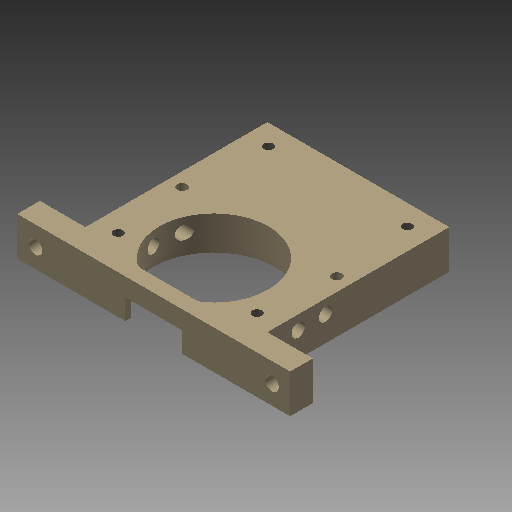
# Autodesk Inventor part: Lichtschranke3
Saved by Autodesk Inventor 2018 (Build 220112000, 112)
## iProperties
Created: 2012-08-13
Part Number: Lichtschranke3
Material: PMMA Plastic
Document SubType Name: Modeling
Designer: Neef
Mass: 81.8294 g
Surface Area: 151.28 cm^2
Volume: 68.88 cm^3
Density: 1.188 g/cm^3
Appearance: Wheat
Author: neef
Autodesk Inventor part; units mm, degrees
ref_plane "YZ Plane" through (0, 0, 0) normal (1, 0, 0) x (0, 1, 0)
ref_plane "XZ Plane" through (0, 0, 0) normal (0, 1, 0) x (-1, 0, 0)
ref_plane "XY Plane" through (0, 0, 0) normal (0, 0, 1) x (1, 0, 0)
sketch "Skizze1" plane through (0, 0, 0) normal (0, 0, 1) x (1, 0, 0)
  line L0 (-40, 45) -> (40, 45)
  line L1 (40, 45) -> (40, -45)
  line L2 (40, -45) -> (-40, -45)
  line L3 (-40, -45) -> (-40, 45)
  line L4 (0, 63) -> (0, -63) projected
  line L5 (-56, 0) -> (56, 0) projected
  point P0 (0, 0)
  point P1 (0, 45)
  point P2 (-40, 0)
  dimension "d0" = 80
  dimension "d1" = 90
  constraints: 8 end point, 2 midpoint, 2 parallel, 2 point on line, 1 horizontal, 1 perpendicular
  measures "d0" distance of L0.start L0.end
  measures "d1" distance of L2.end L0.start
extrude "Extrusion1" add sketch "Skizze1" along normal blind 12
sketch "Skizze2" plane through (0, 0, 0) normal (0, 0, -1) x (-1, 0, 0)
  circle A0 centre (0, -13) radius 5 projected
  circle A1 centre (0, -13) radius 12.5
  point P0 (0, 0)
  dimension "d4" = 25
  constraints: 1 centre point, 1 coincident
  measures "d4" diameter of A1
extrude "Extrusion2" cut sketch "Skizze2" against normal up to surface (12 mm away) contours A0 | A1
sketch "Skizze4" plane through (0, 0, 0) normal (0, 0, -1) x (-1, 0, 0)
  circle A0 centre (30.5, -29.5) radius 2.6 projected
  circle A1 centre (-30.5, -29.5) radius 2.6 projected
  circle A2 centre (30.5, 36.5) radius 2.6 projected
  circle A3 centre (-30.5, 36.5) radius 2.6 projected
  circle A4 centre (-30.5, 36.5) radius 4
  circle A5 centre (30.5, 36.5) radius 4
  circle A6 centre (30.5, -29.5) radius 4
  circle A7 centre (-30.5, -29.5) radius 4
  point P0 (0, 0)
  dimension "d14" = 8
  dimension "d15" = 8
  dimension "d16" = 8
  dimension "d17" = 8
  constraints: 4 centre point, 4 coincident
  measures "d14" diameter of A4
  measures "d15" diameter of A5
  measures "d16" diameter of A6
  measures "d17" diameter of A7
extrude "Extrusion3" cut sketch "Skizze4" against normal blind 4.1
sketch "Skizze6" plane through (0, 0, 0) normal (0, 0, -1) x (-1, 0, 0)
  circle A0 centre (0, -13) radius 12.5 projected
  line L0 (40, 45) -> (40, -45) projected
  arc A1 (0, -29.5) -> (0, 3.5) centre (0, -13) ccw
  arc A2 (19.5, -13) -> (0, 6.5) centre (0, -13) ccw
  line L1 (23.5, -20.5) -> (21, -20.5)
  line L2 (19.5, -13) -> (19.5, -19)
  line L3 (0, 14.2636) -> (0, -32.5)
  line L4 (0, -32.5) -> (20.7123, -32.5)
  line L5 (23.5, -27.0294) -> (23.5, -20.5)
  arc A3 (19.5, -19) -> (21, -20.5) centre (21, -19) ccw
  circle A4 centre (0, -18.5) radius 25 construction
  arc A5 (20.7123, -32.5) -> (23.5, -27.0294) centre (0, -18.5) ccw
  point P0 (0, 0)
  dimension "d22" = 33
  dimension "d23" = 39
  dimension "d24" = 7.5
  dimension "d25" = 19.5
  dimension "d27" = 19.5
  dimension "d28" = 23.5
  dimension "d29" = 1.5
  dimension "d70" = 50
  constraints: 10 end point, 10 point on circle, 5 centre point, 4 point on line, 4 tangent, 3 perpendicular, 2 coincident, 2 parallel, 1 concentric
  measures "d22" diameter of A1
  measures "d23" diameter of A2
  measures "d24" distance from line of A2.centre L1
  measures "d25" distance from line of A0.centre L2
  measures "d27" distance from line of A0.centre L4
  measures "d28" distance from line of A0.centre L5
  measures "d29" radius of A3
  measures "d70" diameter of A4
extrude "Extrusion4" add sketch "Skizze6" along normal blind 5 contours L3 A2 L2 A3 L1 L5 A5 L4 A1
mirror "Spiegeln1" about plane through (0, 3.5, 0) normal (1, 0, 0) of "Extrusion4"
chamfer "Fase1" distance 2 angle 45 1 edges at (0, -29.5, -5)
sketch "Skizze8" plane through (40, -45, 0) normal (1, 0, 0) x (0, 0, -1)
  line L0 (0, 19.5) -> (-12, 19.5) projected
  point P0 (0, 45)
  point P1 (-6, 23.5)
  point P2 (-6, 35.5)
  dimension "d45" = 12
  dimension "d46" = 4
  measures "d45" distance of point (-6, 35.5) point (-6, 23.5)
  measures "d46" distance from line of point (-6, 23.5) L0
hole "Bohrung3" at (40, -21.5, 6) at (40, -9.5, 6) direction (-1, 0, 0) diameter 5.9 end through all
sketch "Skizze11" plane through (0, 0, -5) normal (0, 0, -1) x (-1, 0, 0)
  arc A0 (19.5, -13) -> (-19.5, -13) centre (0, -13) ccw projected
  circle A1 centre (0, -18.5) radius 25
  circle A2 centre (0, -18.5) radius 27
  point P0 (0, 0)
  dimension "d60" = 50
  dimension "d61" = 54
  constraints: 2 centre point, 1 coincident, 1 tangent
  measures "d60" diameter of A1
  measures "d61" diameter of A2
sketch "Skizze12" plane through (0, 0, 0) normal (0, 0, -1) x (-1, 0, 0)
  line L0 (-12.5, -47.3071) -> (12.5, -47.3071)
  line L1 (12.5, -47.3071) -> (12.5, -42)
  line L2 (10.5, -40) -> (-10.5, -40)
  line L3 (-12.5, -42) -> (-12.5, -47.3071)
  line L4 (40, -45) -> (-40, -45) projected
  arc A0 (-10.5, -40) -> (-12.5, -42) centre (-10.5, -42) ccw
  arc A1 (12.5, -42) -> (10.5, -40) centre (10.5, -42) ccw
  point P0 (0, -18.5)
  point P1 (0, 0)
  point P2 (12.5, -40)
  point P3 (-12.5, -40)
  point P4 (5.172, -45)
  dimension "d64" = 25
  dimension "d65" = 12.5
  dimension "d66" = 5
  dimension "d67" = 2
  constraints: 8 end point, 4 point on circle, 4 point on line, 4 tangent, 2 centre point, 2 parallel, 1 equal radius, 1 horizontal, 1 perpendicular
  measures "d64" distance of point (12.5, -40) point (-12.5, -40)
  measures "d65" distance from line of point (0, -18.5) L1
  measures "d66" distance between parallel lines of L2 L4
  measures "d67" radius of A0
extrude "Extrusion8" cut sketch "Skizze11" against normal blind 7.5
extrude "Extrusion9" cut sketch "Skizze12" against normal blind 4
sketch "Skizze13" plane through (0, 0, -5) normal (0, 0, -1) x (-1, 0, 0)
  circle A0 centre (0, -13) radius 18.5 projected
  line L0 (13.2665, -38.5) -> (-13.2665, -38.5)
  arc A1 (11.8422, -40.5173) -> (10.5, -40) centre (10.5, -42) ccw projected
  arc A2 (11.8422, -40.5173) -> (20.7123, -32.5) centre (0, -18.5) ccw projected
  line L1 (20.7123, -32.5) -> (-20.7123, -32.5) projected
  arc A3 (-20.7123, -32.5) -> (-11.8422, -40.5173) centre (0, -18.5) ccw projected
  arc A4 (-10.5, -40) -> (-11.8422, -40.5173) centre (-10.5, -42) ccw projected
  line L2 (-10.5, -40) -> (10.5, -40) projected
  arc A5 (0, 6.5) -> (-23.5, -27.0294) centre (0, -18.5) ccw projected
  line L3 (-23.5, -27.0294) -> (-23.5, -20.5) projected
  line L4 (-23.5, -20.5) -> (-21, -20.5) projected
  arc A6 (-21, -20.5) -> (-19.5, -19) centre (-21, -19) ccw projected
  line L5 (-19.5, -19) -> (-19.5, -13) projected
  arc A7 (0, 6.5) -> (-19.5, -13) centre (0, -13) ccw projected
  arc A8 (23.5, -27.0294) -> (0, 6.5) centre (0, -18.5) ccw projected
  arc A9 (19.5, -13) -> (0, 6.5) centre (0, -13) ccw projected
  line L6 (19.5, -13) -> (19.5, -19) projected
  arc A10 (19.5, -19) -> (21, -20.5) centre (21, -19) ccw projected
  line L7 (21, -20.5) -> (23.5, -20.5) projected
  line L8 (23.5, -20.5) -> (23.5, -27.0294) projected
  arc A11 (13.2665, -38.5) -> (-13.2665, -38.5) centre (0, -18.5) ccw
  point P0 (0, 0)
  dimension "d75" = 1.5
  dimension "d77" = 1
  constraints: 2 end point, 2 point on circle, 1 centre point, 1 coincident
  measures "d75" distance between parallel lines of L0 L2
  measures "d77" radial gap between concentric circles of A5 A11
extrude "Extrusion10" cut sketch "Skizze13" against normal up to surface (17 mm away) contours A0 | A11 A9 L6 A10 L7 L8 L1 L3 L4 A6 L5 A7 | A11 L8 L7 A10 L6 A9 | A7 L5 A6 L4 L3 A11 | A11 L0 L1
sketch "Skizze14" plane through (-40, -45, 12) normal (0, -1, 0) x (1, 0, 0)
  line L0 (0, -12) -> (80, -12)
  line L1 (80, -12) -> (80, -25.8372)
  line L2 (80, -25.8372) -> (0, -25.8372)
  line L3 (0, -25.8372) -> (0, -12)
  point P0 (40, -12)
  constraints: 8 end point, 2 parallel, 1 horizontal, 1 perpendicular
extrude "Extrusion11" cut sketch "Skizze14" against normal up to surface (90 mm away)
fillet "Rundung1" radius 4 2 edges at (-13.2665, -38.5, 6) (13.2665, -38.5, 6)
sketch "Skizze16" plane through (0, 0, 0) normal (0, 0, -1) x (-1, 0, 0)
  circle A0 centre (-30.5, 36.5) radius 4 projected
  circle A1 centre (30.5, -29.5) radius 4 projected
  circle A2 centre (30.5, 36.5) radius 4 projected
  circle A3 centre (-30.5, -29.5) radius 4 projected
  circle A4 centre (-30.5, 36.5) radius 2.6 projected
  circle A5 centre (30.5, 36.5) radius 2.6 projected
  circle A6 centre (30.5, -29.5) radius 2.6 projected
  circle A7 centre (-30.5, -29.5) radius 2.6 projected
  point P0 (0, 0)
extrude "Extrusion13" add sketch "Skizze16" against normal up to surface (4.1 mm away)
sketch "Skizze17" plane through (0, 0, 0) normal (0, 0, -1) x (-1, 0, 0)
  line L0 (12.5, -42.4322) -> (12.5, -45) projected
  line L1 (40, -45) -> (12.5, -45) projected
  line L2 (40, 45) -> (40, -45) projected
  line L3 (-40, 45) -> (40, 45) projected
  line L4 (-40, -45) -> (-40, 45) projected
  line L5 (-12.5, -45) -> (-40, -45) projected
  line L6 (-12.5, -45) -> (-12.5, -42.4322) projected
  arc A0 (12.5, -42.4322) -> (-12.5, -42.4322) centre (0, -18.5) ccw projected
  line L7 (12, -38.5) -> (-12, -38.5) projected
  arc A1 (-14.4, -37.7) -> (-12, -38.5) centre (-12, -34.5) ccw projected
  arc A2 (14.4, -37.7) -> (-14.4, -37.7) centre (0, -18.5) ccw projected
  arc A3 (12, -38.5) -> (14.4, -37.7) centre (12, -34.5) ccw projected
  arc A4 (11.8422, -40.5173) -> (-11.8422, -40.5173) centre (0, -18.5) ccw projected
  arc A5 (-10.5, -40) -> (-11.8422, -40.5173) centre (-10.5, -42) ccw projected
  line L8 (-10.5, -40) -> (10.5, -40) projected
  arc A6 (11.8422, -40.5173) -> (10.5, -40) centre (10.5, -42) ccw projected
  line L9 (40, -39.7) -> (16.72, -39.7)
  line L10 (-16.72, -39.7) -> (-40, -39.7)
  line L11 (12, -38.5) -> (15, -38.5)
  line L12 (18.1384, -38.5) -> (40, -38.5)
  line L13 (-12, -38.5) -> (-15, -38.5)
  line L14 (-18.1384, -38.5) -> (-40, -38.5)
  point P0 (0, 0)
  dimension "d88" = 1.2
  dimension "d112" = 1.2
  constraints: 12 end point, 6 perpendicular, 6 point on circle, 4 point on line, 4 tangent
  measures "d88" distance between parallel lines of L12 L9
  measures "d112" distance between parallel lines of L14 L10
extrude "Extrusion14" add sketch "Skizze17" along normal blind 5 contours A0 L9 L2 L1 L0 | A0 L14 L4 L3 L2 L12 | A0 L6 L5 L4 L10
sketch "Skizze19" plane through (0, 0, 12) normal (0, 0, 1) x (1, 0, 0)
  line L0 (40, -45) -> (-40, -45) projected
  line L1 (40, 45) -> (40, -45) projected
  line L2 (30.5, -30) -> (-30.5, -30) construction
  line L3 (-30.5, -30) -> (-30.5, 36) construction
  line L4 (-30.5, 36) -> (30.5, 36) construction
  line L5 (30.5, 36) -> (30.5, -30) construction
  point P0 (0, 0)
  dimension "d113" = 61
  dimension "d114" = 66
  dimension "d115" = 15
  dimension "d116" = 9.5
  constraints: 8 end point, 4 coincident, 2 parallel, 1 horizontal, 1 perpendicular
  measures "d113" distance of L3.end L4.end
  measures "d114" distance of L2.end L3.end
  measures "d115" distance between parallel lines of L0 L2
  measures "d116" distance between parallel lines of L5 L1
hole "Bohrung4" at (30.5, 36, 12) at (-30.5, 36, 12) at (-30.5, -30, 12) at (30.5, -30, 12) direction (0, 0, -1) diameter 4.134 end through all thread size "M5x0.8" class "6H" standard "ISO Metric profile"
sketch "Skizze20" plane through (-40, -45, 12) normal (0, -1, 0) x (1, 0, 0)
  line L0 (80, 0) -> (100, 0)
  line L1 (100, 0) -> (100, -17)
  line L2 (100, -17) -> (80, -17)
  line L3 (80, -17) -> (80, 0)
  point P0 (40, -12)
  dimension "d124" = 20
  dimension "d125" = 17
  constraints: 8 end point, 2 parallel, 1 horizontal, 1 perpendicular
  measures "d124" distance of L0.start L0.end
  measures "d125" distance of L0.end L1.end
extrude "Extrusion17" add sketch "Skizze20" against normal blind 10
sketch "Skizze21" plane through (-40, -35, 12) normal (0, 1, 0) x (1, 0, 0)
  line L0 (100, 17) -> (100, 0) projected
  point P0 (40, 12)
  point P1 (92, 8.5)
  dimension "d128" = 8
  measures "d128" distance from line of L0 point (92, 8.5)
hole "Bohrung5" at (52, -35, 3.5) direction (0, -1, 0) diameter 6 end through all
mirror "Spiegeln2" about plane through (0, 0, 0) normal (1, 0, 0) of "Extrusion17", "Bohrung5"
move faces "Fläche verschieben3" translate (-20, 0, 0) faces at (-40, -39.3, -1.6667)
sketch "Skizze22" plane through (0, 0, 12) normal (0, 0, 1) x (1, 0, 0)
  line L0 (-40, -35) -> (-40, 45) projected
  line L1 (-60, -45) -> (60, -45) projected
  circle A0 centre (-34, 1.5) radius 1.621 projected
  point P0 (0, 0)
  point P1 (-34, 1.5)
  dimension "d136" = 6
  dimension "d137" = 46.5
  measures "d136" distance from line of L0 point (-34, 1.5)
  measures "d137" distance from line of point (-34, 1.5) L1
hole "Bohrung6" at (-34, 1.5, 12) direction (0, 0, -1) diameter 4.4 end up to surface
mirror "Spiegeln3" about plane through (0, 0, 0) normal (1, 0, 0) of "Bohrung6"
equation "\"d65\" = 0.5 * d64"
equation "\"d112\" = d88"
